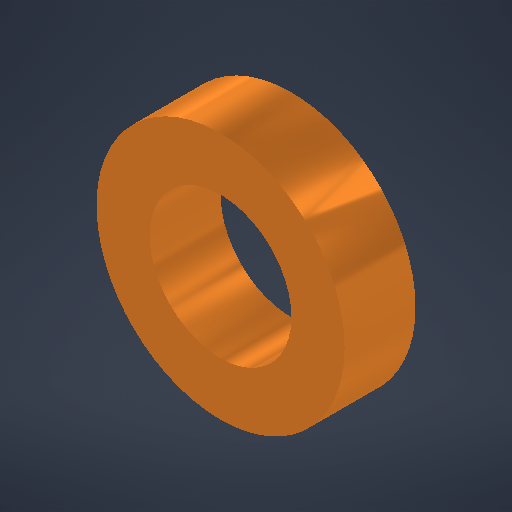
# Autodesk Inventor part: bearing_mass
Saved by Autodesk Inventor 2026 (Build 300175000, 175)
## iProperties
Created: 2026-04-27
Part Number: bearing_mass
Material: Золото
Document SubType Name: Modeling
Designer: user
Density: 78.4 g/cm^3
Appearance: Металл — 1600F
Mass: 507.996 g
Surface Area: 30.2378 cm^2
Volume: 6.47953 cm^3
Author: user
Autodesk Inventor part; units mm, degrees
ref_plane "YZ Plane" through (0, 0, 0) normal (1, 0, 0) x (0, 1, 0)
ref_plane "XZ Plane" through (0, 0, 0) normal (0, 1, 0) x (-1, 0, 0)
ref_plane "XY Plane" through (0, 0, 0) normal (0, 0, 1) x (1, 0, 0)
sketch "Эскиз1" plane through (0, 0, 0) normal (0, 0, 1) x (1, 0, 0)
  circle A0 centre (0, 0) radius 10
  circle A1 centre (0, 0) radius 17.5
  dimension "d0" = 20
  dimension "d1" = 35
  constraints: 2 centre point, 2 coincident
  measures "d0" diameter of A0
  measures "d1" diameter of A1
extrude "Выдавливание1" add sketch "Эскиз1" along normal blind 10
equation "\"d0\" = d_main_shaft"
equation "\"tolerance_plazma\" = 0.1"
equation "\"thickness_steel\" = 3"
equation "\"d_main_screw_holes\" = 6.1"
equation "\"d_main_shaft\" = 20"
equation "\"width_flattened_surface\" = 12"
equation "\"thickness_profile_tibea\" = 4"
equation "\"thickness_profile_femur\" = 3"
equation "\"width_shaft_shift\" = 35"
